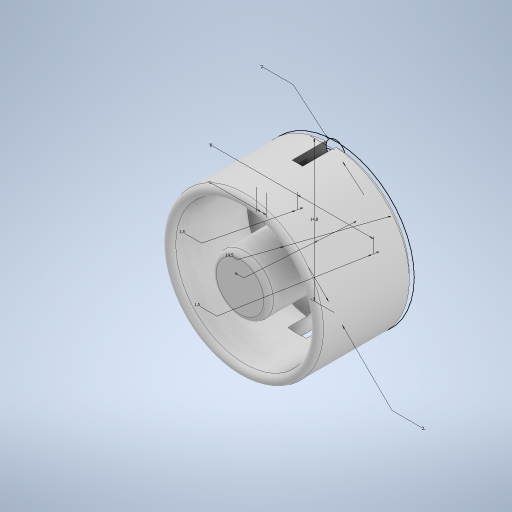
# Autodesk Inventor part: ATU_T50_SUPPORT
Saved by Autodesk Inventor 2024 (Build 280153000, 153)
## iProperties
Created: 2025-01-31
Part Number: ATU_T50_SUPPORT
Material: Типовые
Document SubType Name: Modeling
Designer: fm
Density: 1 g/cm^3
Appearance: По умолчанию
Author: fm
Autodesk Inventor part; units mm, degrees
ref_plane "YZ Plane" through (0, 0, 0) normal (1, 0, 0) x (0, 1, 0)
ref_plane "XZ Plane" through (0, 0, 0) normal (0, 1, 0) x (-1, 0, 0)
ref_plane "XY Plane" through (0, 0, 0) normal (0, 0, 1) x (1, 0, 0)
sketch "Эскиз1" plane through (0, 0, 0) normal (0, 0, 1) x (1, 0, 0)
  circle A0 centre (0, 0) radius 3
  circle A1 centre (0, 0) radius 7.25
  circle A2 centre (0, 0) radius 8.25
  circle A3 centre (-4, 0) radius 0.75
  line L0 (-4, 0) -> (4, 0)
  circle A4 centre (4, 0) radius 0.75
  line L1 (0, 7.4) -> (0, -7.4)
  circle A5 centre (0, 7.4) radius 1
  circle A6 centre (0, -7.4) radius 1
  dimension "d0" = 6
  dimension "d1" = 14.5
  dimension "d2" = 1
  dimension "d3" = 1.5
  dimension "d4" = 8
  dimension "d5" = 1.5
  dimension "d19" = 14.8
  dimension "d20" = 2
  dimension "d21" = 2
  constraints: 7 centre point, 6 coincident, 4 end point, 2 midpoint, 1 horizontal, 1 vertical
  measures "d0" diameter of A0
  measures "d1" diameter of A1
  measures "d2" radial gap between concentric circles of A1 A2
  measures "d3" diameter of A3
  measures "d4" distance of L0.start L0.end
  measures "d5" diameter of A4
  measures "d19" distance of L1.start L1.end
  measures "d20" diameter of A5
  measures "d21" diameter of A6
extrude "Выдавливание1" add sketch "Эскиз1" along normal blind 2 contours L0 L1 A0 | A0 L1 A5 A1 A6 | A0 L1 L0 | L1 L0 A0 | A0 L1 A6 A1 A5 | A0 L0 L1 | A5 A1 L1 | L1 A1 A5 | A6 A1 L1 | L1 A1 A6 | A1 A5 A2 | A1 A6 A2 A5 | A5 A2 A6 A1 | A1 A6 A2 | A3 | A4
extrude "Выдавливание2" add sketch "Эскиз1" along normal blind 8 from surface at 2 contours L0 L1 A0 | A0 L1 L0 | L1 L0 A0 | A0 L0 L1 | A1 A5 A2 | A1 A6 A2 A5 | A5 A2 A6 A1 | A1 A6 A2
extrude "Выдавливание3" cut sketch "Эскиз1" along normal through all contours A3 | A4
chamfer "Фаска1" distance 1 angle 45 2 edges at (-4.75, 0, 2) (3.25, 0, 2)
fillet "Сопряжение1" radius 0.5 3 edges at (-3, 0, 10) (-7.25, 0, 10) (-8.25, 0, 10)
chamfer "Фаска2" distance 0.5 angle 45 1 edges at (-8.25, 0, 0)
extrude "Выдавливание4" cut sketch "Эскиз1" along normal blind 4 contours A5 A1 L1 | L1 A1 A5 | A6 A1 L1 | L1 A1 A6 | A1 A5 A2 | A1 A6 A2 | A5 A2 | A2 A6
